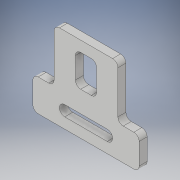
# Autodesk Inventor part: P2-7
Saved by Autodesk Inventor 2017 (Build 210142000, 142)
## iProperties
Created: 2017-02-09
Part Number: P2-7
Material: Generic
Document SubType Name: Modeling
Designer: Schaffel
Density: 1 g/cm^3
Appearance: Default
Author: Schaffel
Autodesk Inventor part; units mm, degrees
ref_plane "YZ Plane" through (0, 0, 0) normal (1, 0, 0) x (0, 1, 0)
ref_plane "XZ Plane" through (0, 0, 0) normal (0, 1, 0) x (-1, 0, 0)
ref_plane "XY Plane" through (0, 0, 0) normal (0, 0, 1) x (1, 0, 0)
sketch "Sketch1" plane through (0, 0, 0) normal (0, 0, 1) x (1, 0, 0)
  line L0 (6.35, 0) -> (120.65, 0)
  line L1 (127, 6.35) -> (127, 31.75)
  line L2 (120.65, 38.1) -> (107.95, 38.1)
  line L3 (101.6, 44.45) -> (101.6, 95.25)
  line L4 (95.25, 101.6) -> (31.75, 101.6)
  line L5 (25.4, 95.25) -> (25.4, 44.45)
  line L6 (19.05, 38.1) -> (6.35, 38.1)
  line L7 (0, 31.75) -> (0, 6.35)
  arc A0 (31.75, 101.6) -> (25.4, 95.25) centre (31.75, 95.25) ccw
  arc A1 (19.05, 38.1) -> (25.4, 44.45) centre (19.05, 44.45) ccw
  arc A2 (6.35, 38.1) -> (0, 31.75) centre (6.35, 31.75) ccw
  arc A3 (0, 6.35) -> (6.35, 0) centre (6.35, 6.35) ccw
  arc A4 (120.65, 0) -> (127, 6.35) centre (120.65, 6.35) ccw
  arc A5 (127, 31.75) -> (120.65, 38.1) centre (120.65, 31.75) ccw
  arc A6 (101.6, 44.45) -> (107.95, 38.1) centre (107.95, 44.45) ccw
  arc A7 (101.6, 95.25) -> (95.25, 101.6) centre (95.25, 95.25) ccw
  line L8 (57.15, 50.8) -> (69.85, 50.8)
  line L9 (76.2, 57.15) -> (76.2, 82.55)
  line L10 (69.85, 88.9) -> (57.15, 88.9)
  line L11 (50.8, 82.55) -> (50.8, 57.15)
  arc A8 (38.1, 25.4) -> (38.1, 12.7) centre (38.1, 19.05) ccw
  arc A9 (88.9, 12.7) -> (88.9, 25.4) centre (88.9, 19.05) ccw
  line L12 (38.1, 25.4) -> (88.9, 25.4)
  line L13 (88.9, 12.7) -> (38.1, 12.7)
  arc A10 (57.15, 88.9) -> (50.8, 82.55) centre (57.15, 82.55) ccw
  arc A11 (50.8, 57.15) -> (57.15, 50.8) centre (57.15, 57.15) ccw
  arc A12 (69.85, 50.8) -> (76.2, 57.15) centre (69.85, 57.15) ccw
  arc A13 (76.2, 82.55) -> (69.85, 88.9) centre (69.85, 82.55) ccw
  point P0 (0, 0)
  point P1 (127, 0)
  point P2 (127, 38.1)
  point P3 (101.6, 38.1)
  point P4 (25.4, 38.1)
  point P5 (0, 38.1)
  dimension "d0" = 127
  dimension "d1" = 38.1
  dimension "d2" = 25.4
  dimension "d3" = 6.35
  dimension "d4" = 6.35
  constraints: 28 end point, 28 point on circle, 24 tangent, 14 centre point, 14 point on line, 10 equal radius, 8 perpendicular, 3 horizontal, 1 parallel
  measures "d0" distance of point (0, 0) point (127, 0)
  measures "d1" distance of point (127, 0) point (127, 38.1)
  measures "d2" distance of point (127, 38.1) point (101.6, 38.1)
  measures "d3" radius of A0
  measures "d4" radius of A10
extrude "Extrusion1" add sketch "Sketch1" along normal blind 9.525
body "Solid1"
